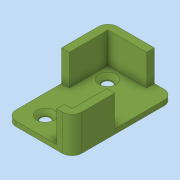
# Autodesk Inventor part: limitSwitchHolder2
Saved by Autodesk Inventor 2017 (Build 210142000, 142)
## iProperties
Created: 2016-12-04
Part Number: limitSwitchHolder2
Material: ABS Plastic
Document SubType Name: Modeling
Designer: techn
Density: 1.06 g/cm^3
Appearance: Olive Green
Author: techn
Autodesk Inventor part; units mm, degrees
ref_plane "YZ Plane" through (0, 0, 0) normal (1, 0, 0) x (0, 1, 0)
ref_plane "XZ Plane" through (0, 0, 0) normal (0, 1, 0) x (-1, 0, 0)
ref_plane "XY Plane" through (0, 0, 0) normal (0, 0, 1) x (1, 0, 0)
sketch "Sketch2" plane through (0, 0, 0) normal (0, 1, 0) x (-1, 0, 0)
  line L0 (0, 0) -> (2.54, 0)
  line L1 (2.54, 0) -> (2.54, 2.54)
  line L2 (2.54, 2.54) -> (0, 2.54)
  line L3 (0, 2.54) -> (0, 0)
  line L4 (0, 0) -> (-2.54, 0)
  line L5 (-2.54, 0) -> (-2.54, -11.43)
  line L6 (-2.54, -11.43) -> (0, -11.43)
  line L7 (0, -11.43) -> (0, 0)
  line L8 (-2.54, 0) -> (0, 0)
  line L9 (0, 0) -> (0, 2.54)
  line L10 (0, 2.54) -> (-2.54, 2.54)
  line L11 (-2.54, 2.54) -> (-2.54, 0)
  line L12 (16.51, -15.621) -> (19.05, -15.621)
  line L13 (19.05, -15.621) -> (19.05, -28.321)
  line L14 (19.05, -28.321) -> (16.51, -28.321)
  line L15 (16.51, -28.321) -> (16.51, -15.621)
  line L16 (19.05, -28.321) -> (3.81, -28.321)
  line L17 (3.81, -28.321) -> (3.81, -30.861)
  line L18 (3.81, -30.861) -> (19.05, -30.861)
  line L19 (19.05, -30.861) -> (19.05, -28.321)
  line L20 (19.05, -30.861) -> (-2.54, -30.861)
  line L21 (-2.54, -30.861) -> (-2.54, 2.54)
  line L22 (-2.54, 2.54) -> (19.05, 2.54)
  line L23 (19.05, 2.54) -> (19.05, -30.861)
  line L24 (0, 0) -> (2.54, 0)
  line L25 (2.54, 0) -> (2.54, 2.54)
  line L26 (2.54, 2.54) -> (0, 2.54)
  line L27 (0, 2.54) -> (0, 0)
  line L28 (-2.54, -11.43) -> (0, -11.43)
  line L29 (0, -11.43) -> (0, 2.54)
  line L30 (0, 2.54) -> (-2.54, 2.54)
  line L31 (-2.54, 2.54) -> (-2.54, -11.43)
  dimension "d0" = 2.54
  dimension "d1" = 2.54
  dimension "d2" = 2.54
  dimension "d3" = 11.43
  dimension "d4" = 2.54
  dimension "d5" = 12.7
  dimension "d6" = 15.24
  dimension "d7" = 2.54
  dimension "d8" = 16.51
  dimension "d9" = 28.321
  constraints: 64 end point, 16 parallel, 8 horizontal, 8 perpendicular
  measures "d0" distance of L2.end L1.end
  measures "d1" distance of L1.end L0.end
  measures "d2" distance of L6.end L5.end
  measures "d3" distance of L5.end L4.end
  measures "d4" distance of L13.end L14.end
  measures "d5" distance of L12.end L13.end
  measures "d6" distance of L18.end L17.end
  measures "d7" distance of L17.end L16.end
  measures "d8" distance between parallel lines of L15 L7
  measures "d9" distance between parallel lines of L16 L0
extrude "Extrusion1" add sketch "Sketch2" along normal blind 10.16 contours L3 L2 L1 L0 | L4 L11 L10 L3 | L7 L6 L5 L4 | L13 L14 L15 L12 | L17 L16 L14 L19 L18
extrude "Extrusion2" add sketch "Sketch2" against normal blind 1.5875
sketch "Sketch4" plane through (0, 0, 0) normal (0, 1, 0) x (1, 0, 0)
  circle A0 centre (-12.7, 3.9624) radius 1.5875
  circle A1 centre (-12.7, 24.3586) radius 1.5875
  line L0 (-19.05, 15.621) -> (-19.05, -2.54) projected
  line L1 (-19.05, -2.54) -> (-2.54, -2.54) projected
  line L2 (2.54, 30.861) -> (-3.81, 30.861) projected
  point P0 (0, 0)
  dimension "d14" = 3.175
  dimension "d15" = 3.175
  dimension "d16" = 6.35
  dimension "d17" = 6.35
  dimension "d23" = 20.3962
  dimension "d24" = 6.5024
  dimension "d25" = 33.401
  constraints: 2 centre point
  measures "d14" diameter of A0
  measures "d15" diameter of A1
  measures "d16" distance from line of L0 A0.centre
  measures "d17" distance from line of L0 A1.centre
  measures "d23" distance of A1.centre A0.centre
  measures "d24" distance from line of L2 A1.centre
  measures "d25" distance between parallel lines of L1 L2
extrude "Extrusion3" cut sketch "Sketch4" against normal blind 1.5875
fillet "Fillet1" radius 3.175 4 edges at (2.54, -0.7937, -30.861) (2.54, 4.2862, 2.54) (-19.05, -0.7937, 2.54) (-19.05, 4.2863, -30.861)
chamfer "Chamfer1" distance 1.27 angle 45 2 edges at (-14.2875, 0, -24.3586) (-14.2875, 0, -3.9624)
equation "\"d24\" = -0.5 * d23 + 0.5 * d25"
body "Solid1"
